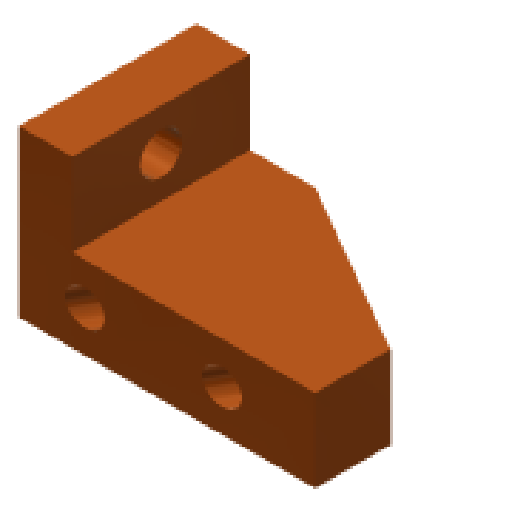
# Autodesk Inventor part: LEDBracket
Saved by Autodesk Inventor 2023.2 (Build 272271000, 271)
## iProperties
Created: 2021-03-28
Part Number: LEDBracket
Material: ABS Plastic
Document SubType Name: Modeling
Designer: Remo
Mass: 1.41087 g
Surface Area: 11.1875 cm^2
Volume: 1.50092 cm^3
Density: 1.06 g/cm^3
Appearance: Smooth - Light Orange
Author: Remo
Autodesk Inventor part; units mm, degrees
ref_plane "YZ Plane" through (0, 0, 0) normal (1, 0, 0) x (0, 1, 0)
ref_plane "XZ Plane" through (0, 0, 0) normal (0, 1, 0) x (-1, 0, 0)
ref_plane "XY Plane" through (0, 0, 0) normal (0, 0, 1) x (1, 0, 0)
sketch "Sketch1" plane through (0, 0, 0) normal (0, 1, 0) x (-1, 0, 0)
  line L0 (0, 0) -> (0, -6.3397)
  line L1 (0, -6.3397) -> (15, -15)
  line L2 (25, 0) -> (0, 0)
  line L3 (25, 0) -> (25, -15)
  line L4 (25, -15) -> (15, -15)
  dimension "d1" = 60
  dimension "d25" = 15
  dimension "d26" = 10
  dimension "d27" = 15
  constraints: 10 end point, 2 vertical, 1 horizontal, 1 perpendicular
  measures "d1" angle of L1 L0
  measures "d25" distance of L2.start L3.end
  measures "d26" distance of L3.end L1.end
  measures "d27" distance from line of L1.end L0
extrude "Extrusion1" add sketch "Sketch1" along normal blind 7
sketch "Sketch2" plane through (-15, 0, -15) normal (0.5, 0, -0.866) x (-0.866, 0, -0.5)
  line L0 (-17.3205, 0) -> (0, 0) projected
  line L1 (0, 0) -> (0, 7) projected
  line L2 (-17.3205, 7) -> (0, 7) projected
  line L3 (-17.3205, 0) -> (-17.3205, 7) projected
  circle A0 centre (-3.6603, 3.5) radius 1.45
  circle A1 centre (-13.6603, 3.5) radius 1.45
  point P0 (-20.4904, 0)
  dimension "d5" = 2.9
  dimension "d6" = 10
  dimension "d8" = 7
  dimension "d9" = 3.5
  dimension "d10" = 17.3205
  dimension "d11" = 3.6603
  constraints: 2 centre point, 1 equal radius, 1 horizontal alignment
  measures "d5" diameter of A0
  measures "d6" distance of A1.centre A0.centre
  measures "d8" distance between parallel lines of L2 L0
  measures "d9" distance from line of L2 A1.centre
  measures "d10" distance of L0.start L0.end
  measures "d11" distance from line of L3 A1.centre
extrude "Extrusion2" cut sketch "Sketch2" against normal through all contours A0 | A1
sketch "Sketch6" plane through (0, 7, 0) normal (0, 1, 0) x (1, 0, 0)
  line L0 (0, 0) -> (0, 6.3397) projected
  line L1 (0, 6.3397) -> (-15, 15) projected
  line L2 (-15, 15) -> (-25, 15) projected
  line L3 (-25, 15) -> (-25, 0) projected
  line L4 (-25, 0) -> (0, 0) projected
  line L5 (0, 6.3397) -> (-15, 15) projected
  line L6 (-25, 0) -> (0, 0) projected
  line L7 (-20.5, 15) -> (-20.5, 0)
  dimension "d34" = 4.5
  constraints: 2 end point, 2 point on line, 1 perpendicular
  measures "d34" distance between parallel lines of L3 L7
extrude "Extrusion5" add sketch "Sketch6" along normal blind 7 contours L4 L3 L2 L7
sketch "Sketch8" plane through (-20.5, 7, 0) normal (1, 0, 0) x (0, 0, -1)
  line L0 (15, 0) -> (0, 0) projected
  line L1 (15, 0) -> (15, 7) projected
  line L2 (0, 7) -> (15, 7) projected
  line L3 (0, 0) -> (0, 7) projected
  circle A0 centre (7.5, 3.5) radius 1.75
  point P0 (0, -7)
  point P1 (0, 3.5)
  point P2 (7.5, 0)
  dimension "d35" = 3.5
  constraints: 2 midpoint, 1 centre point, 1 horizontal alignment, 1 vertical alignment
  measures "d35" diameter of A0
extrude "Extrusion7" cut sketch "Sketch8" against normal through all contours A0
equation "\"d9\" = 0.5 * d8"
equation "\"d11\" = -0.5 * d6 + 0.5 * d10"
body "Solid1"
